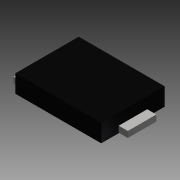
# Autodesk Inventor part: s20A 60V Diode
Saved by Autodesk Inventor 2015 (Build 190159000, 159)
## iProperties
Created: 2016-01-19
Part Number: s20A 60V Diode
Material: Generic
Document SubType Name: Modeling
Designer: Kyle
Density: 1 g/cm^3
Appearance: Default
Author: Kyle
Autodesk Inventor part; units mm, degrees
ref_plane "YZ Plane" through (0, 0, 0) normal (1, 0, 0) x (0, 1, 0)
ref_plane "XZ Plane" through (0, 0, 0) normal (0, 1, 0) x (-1, 0, 0)
ref_plane "XY Plane" through (0, 0, 0) normal (0, 0, 1) x (1, 0, 0)
sketch "Sketch1" plane through (0, 0, 0) normal (0, 0, 1) x (1, 0, 0)
  line L0 (0, 0) -> (5.3696, 0)
  line L1 (5.3696, 0) -> (5.3696, 1.0998)
  line L2 (5.3696, 1.0998) -> (0, 1.0998)
  line L3 (0, 1.0998) -> (0, 0)
  dimension "d0" = 1.0998
  dimension "d1" = 5.3696
  constraints: 8 end point, 2 parallel, 1 horizontal, 1 perpendicular
  measures "d0" distance of L0.end L1.end
  measures "d1" distance of L1.end L2.end
extrude "Extrusion1" add sketch "Sketch1" along normal blind 3.9649
sketch "Sketch2" plane through (5.3696, 0, 0) normal (1, 0, 0) x (0, 0, -1)
  line L0 (-2.8727, 0.4064) -> (-1.0922, 0.4064)
  line L1 (-1.0922, 0.4064) -> (-1.0922, 0.0254)
  line L2 (-1.0922, 0.0254) -> (-2.8727, 0.0254)
  line L3 (-2.8727, 0.0254) -> (-2.8727, 0.4064)
  line L4 (-3.9649, 0) -> (-3.9649, 1.0998) projected
  line L5 (0, 0) -> (-3.9649, 0) projected
  dimension "d4" = 1.7805
  dimension "d5" = 0.381
  dimension "d6" = 1.0922
  dimension "d7" = 0.0254
  constraints: 8 end point, 2 parallel, 1 horizontal, 1 perpendicular
  measures "d4" distance of L1.end L2.end
  measures "d5" distance of L0.end L1.end
  measures "d6" distance between parallel lines of L4 L3
  measures "d7" distance between parallel lines of L2 L5
extrude "Extrusion2" add sketch "Sketch2" along normal blind 0.569
sketch "Sketch3" plane through (0, 0, 0) normal (-1, 0, 0) x (0, 0, 1)
  line L0 (0.4572, 0.4064) -> (1.3462, 0.4064)
  line L1 (1.3462, 0.4064) -> (1.3462, 0.0254)
  line L2 (1.3462, 0.0254) -> (0.4572, 0.0254)
  line L3 (0.4572, 0.0254) -> (0.4572, 0.4064)
  line L4 (2.6187, 0.4064) -> (3.5077, 0.4064)
  line L5 (3.5077, 0.4064) -> (3.5077, 0.0254)
  line L6 (3.5077, 0.0254) -> (2.6187, 0.0254)
  line L7 (2.6187, 0.0254) -> (2.6187, 0.4064)
  line L8 (0, 0) -> (3.9649, 0) projected
  line L9 (0, 1.0998) -> (0, 0) projected
  line L10 (3.9649, 1.0998) -> (3.9649, 0) projected
  dimension "d10" = 0.381
  dimension "d11" = 0.0254
  dimension "d12" = 0.889
  dimension "d13" = 0.889
  dimension "d14" = 0.4572
  dimension "d15" = 0.4572
  constraints: 16 end point, 4 parallel, 2 horizontal, 2 perpendicular, 2 point on line
  measures "d10" distance between parallel lines of L0 L2
  measures "d11" distance between parallel lines of L8 L2
  measures "d12" distance of L0.start L0.end
  measures "d13" distance of L4.start L4.end
  measures "d14" distance between parallel lines of L9 L3
  measures "d15" distance between parallel lines of L10 L5
extrude "Extrusion3" add sketch "Sketch3" along normal blind 0.569
body "Solid1"
